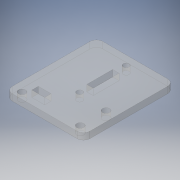
# Autodesk Inventor part: Belt_Holder1
Saved by Autodesk Inventor 2016 (Build 200138000, 138)
## iProperties
Created: 2018-05-31
Part Number: Belt_Holder1
Material: Polycarbonate, Clear
Document SubType Name: Modeling
Designer: Phil Erle
Density: 1.2 g/cm^3
Appearance: Polycarbonate - Clear
Author: Phil Erle
Autodesk Inventor part; units mm, degrees
ref_plane "YZ Plane" through (0, 0, 0) normal (1, 0, 0) x (0, 1, 0)
ref_plane "XZ Plane" through (0, 0, 0) normal (0, 1, 0) x (-1, 0, 0)
ref_plane "XY Plane" through (0, 0, 0) normal (0, 0, 1) x (1, 0, 0)
sketch "Sketch1" plane through (0, 0, 0) normal (0, 0, 1) x (1, 0, 0)
  line L0 (-25, -35) -> (25, -35)
  line L1 (30, -30) -> (30, 30)
  line L2 (25, 35) -> (-25, 35)
  line L3 (-30, 30) -> (-30, -30)
  line L4 (-30, -35) -> (30, 35) construction
  line L5 (30, -35) -> (-30, 35) construction
  arc A0 (-25, 35) -> (-30, 30) centre (-25, 30) ccw
  arc A1 (30, 30) -> (25, 35) centre (25, 30) ccw
  arc A2 (25, -35) -> (30, -30) centre (25, -30) ccw
  arc A3 (-30, -30) -> (-25, -35) centre (-25, -30) ccw
  point P0 (0, 0)
  dimension "d0" = 60
  dimension "d1" = 70
  dimension "d4" = 5
  constraints: 12 end point, 8 point on circle, 8 point on line, 8 tangent, 4 centre point, 3 equal radius, 2 midpoint, 2 parallel, 1 horizontal, 1 perpendicular
  measures "d0" distance of L5.end L4.end
  measures "d1" distance of L4.end L5.start
  measures "d4" radius of A0
extrude "Extrusion1" add sketch "Sketch1" along normal blind 5
sketch "Sketch2" plane through (0, 0, 5) normal (0, 0, 1) x (1, 0, 0)
  line L0 (-22.5, -30.0466) -> (22.5, -30.0466) construction
  line L1 (22.5, -30.0466) -> (22.5, -10.0466) construction
  line L2 (22.5, -10.0466) -> (-22.5, -10.0466) construction
  line L3 (-22.5, -10.0466) -> (-22.5, -30.0466) construction
  line L4 (-22.5, -30.0466) -> (22.5, -10.0466) construction
  line L5 (22.5, -30.0466) -> (-22.5, -10.0466) construction
  point P0 (0, 0)
  point P1 (0, -20.0466)
  point P2 (0, -20.0466)
  dimension "d5" = 45
  dimension "d6" = 20.0466
  dimension "d7" = 20
  constraints: 12 end point, 3 coincident, 3 midpoint, 2 parallel, 1 horizontal, 1 perpendicular, 1 vertical alignment
  measures "d5" distance of L0.start L0.end
  measures "d6" distance of point (0, 0) point (0, -20.047)
  measures "d7" distance of L2.end L0.start
hole "Hole1" at (22.5, -10.0466, 5) at (22.5, -30.0466, 5) at (-22.5, -30.0466, 5) direction (0, 0, -1) diameter 5.5 depth 8 tip angle 118 clearance for "Countersunk Flat Head Screw DIN EN ISO 2009" size "M5" standard "DIN"
sketch "Sketch3" plane through (0, 0, 5) normal (0, 0, 1) x (1, 0, 0)
  line L0 (-2.5, 0) -> (2.5, 0)
  line L1 (2.5, 0) -> (2.5, 20)
  line L2 (2.5, 20) -> (-2.5, 20)
  line L3 (-2.5, 20) -> (-2.5, 0)
  line L4 (-2.5, 0) -> (2.5, 20) construction
  line L5 (2.5, 0) -> (-2.5, 20) construction
  point P0 (0, 0)
  point P1 (0, 10)
  point P2 (0, 10)
  point P3 (0, 0)
  point P4 (0, 10)
  dimension "d15" = 5
  dimension "d16" = 20
  dimension "d17" = 10
  constraints: 12 end point, 5 midpoint, 2 parallel, 2 vertical alignment, 1 horizontal, 1 perpendicular
  measures "d15" distance of L2.end L1.end
  measures "d16" distance of L1.end L0.end
  measures "d17" distance of point (0, 0) point (0, 10)
extrude "Extrusion2" cut sketch "Sketch3" against normal blind 5
sketch "Sketch4" plane through (0, 0, 5) normal (0, 0, 1) x (1, 0, 0)
  line L0 (-2.5, 20) -> (2.5, 20) projected
  line L1 (2.5, 0) -> (-2.5, 0) projected
  point P0 (0, 0)
  point P1 (0, 28)
  point P2 (0, -8)
  point P3 (0, 0)
  dimension "d20" = 8
  dimension "d21" = 8
  constraints: 2 vertical alignment, 1 midpoint
  measures "d20" distance from line of point (0, 28) L0
  measures "d21" distance from line of L1 point (0, -8)
hole "Hole2" at (0, 28, 5) at (0, -8, 5) direction (0, 0, -1) diameter 4.5 depth 8 tip angle 118 clearance for "Countersunk Flat Head Screw DIN EN ISO 2009" size "M4" standard "DIN"
sketch "Sketch5" plane through (0, 0, 5) normal (0, 0, 1) x (1, 0, 0)
  line L0 (2.5, 0) -> (-2.5, 0) projected
  line L1 (-20, -25) -> (-10, -25)
  line L2 (-10, -25) -> (-10, -20)
  line L3 (-10, -20) -> (-20, -20)
  line L4 (-20, -20) -> (-20, -25)
  line L5 (-20, -25) -> (-10, -20) construction
  line L6 (-10, -25) -> (-20, -20) construction
  line L7 (-25, -35) -> (25, -35) projected
  line L8 (-30, 30) -> (-30, -30) projected
  point P0 (0, 0)
  point P1 (0, 0)
  point P2 (-15, -22.5)
  dimension "d34" = 10
  dimension "d35" = 5
  dimension "d36" = 10
  dimension "d37" = 30
  dimension "d38" = 10
  constraints: 12 end point, 3 midpoint, 2 parallel, 1 horizontal, 1 perpendicular
  measures "d34" distance of L2.end L3.end
  measures "d35" distance of L1.end L2.end
  measures "d36" distance between parallel lines of L7 L1
  measures "d37" distance from line of point (0, 0) L8
  measures "d38" distance between parallel lines of L8 L4
extrude "Extrusion3" cut sketch "Sketch5" against normal blind 5
equation "\"d38\" = -0.5 * d34 + 0.5 * d37"
body "Solid1"
